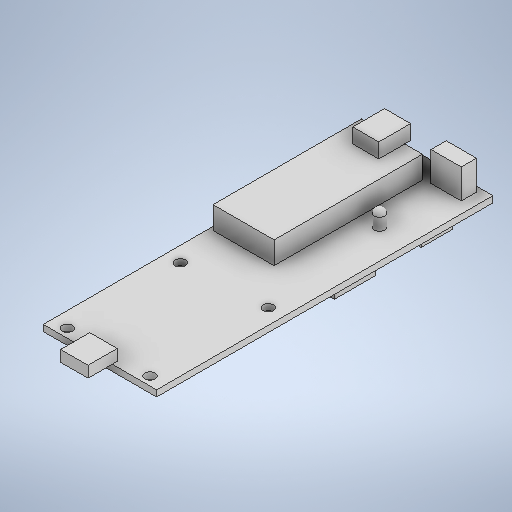
# Autodesk Inventor part: PCB Board
Saved by Autodesk Inventor 2025 (Build 290162000, 162)
## iProperties
Created: 2024-07-09
Part Number: PCB Board
Material: Generic
Document SubType Name: Modeling
Designer: track
Density: 1 g/cm^3
Appearance: Default
Author: track
Autodesk Inventor part; units mm, degrees
ref_plane "YZ Plane" through (0, 0, 0) normal (1, 0, 0) x (0, 1, 0)
ref_plane "XZ Plane" through (0, 0, 0) normal (0, 1, 0) x (-1, 0, 0)
ref_plane "XY Plane" through (0, 0, 0) normal (0, 0, 1) x (1, 0, 0)
sketch "Sketch1" plane through (0, 0, 0) normal (0, 1, 0) x (-1, 0, 0)
  line L0 (16.375, 48.6) -> (-16.375, 48.6)
  line L1 (-16.375, 48.6) -> (-16.375, -48.6)
  line L2 (-16.375, -48.6) -> (16.375, -48.6)
  line L3 (16.375, -48.6) -> (16.375, 48.6)
  line L4 (16.375, 48.6) -> (-16.375, -48.6) construction
  line L5 (-16.375, 48.6) -> (16.375, -48.6) construction
  point P0 (0, 0)
  dimension "d0" = 32.75
  dimension "d1" = 97.2
  constraints: 12 end point, 2 midpoint, 2 parallel, 1 horizontal, 1 perpendicular
  measures "d0" distance of L0.start L0.end
  measures "d1" distance of L0.end L1.end
extrude "Extrusion1" add sketch "Sketch1" along normal blind 1.8
sketch "Sketch4" plane through (0, 0, 0) normal (0, -1, 0) x (1, 0, 0)
  line L0 (8.375, 33.45) -> (-9.375, 33.45)
  line L1 (-9.375, 33.45) -> (-9.375, 15.45)
  line L2 (-9.375, 15.45) -> (8.375, 15.45)
  line L3 (8.375, 15.45) -> (8.375, 33.45)
  line L4 (16.375, 48.6) -> (16.375, -48.6) projected
  line L5 (-16.375, 48.6) -> (16.375, 48.6) projected
  point P0 (0, 0)
  dimension "d12" = 18
  dimension "d13" = 17.75
  dimension "d14" = 8
  dimension "d15" = 15.15
  constraints: 8 end point, 2 parallel, 1 horizontal, 1 perpendicular
  measures "d12" distance of L2.end L0.start
  measures "d13" distance of L1.end L2.end
  measures "d14" distance between parallel lines of L4 L3
  measures "d15" distance between parallel lines of L5 L0
extrude "Extrusion4" add sketch "Sketch4" along normal blind 3.43 from surface at -1.8
sketch "Sketch5" plane through (-9.375, -1.63, 33.45) normal (0, -1, 0) x (1, 0, 0)
  line L0 (2, -9) -> (15.8, -9)
  line L1 (15.8, -9) -> (15.8, 9.6)
  line L2 (15.8, 9.6) -> (2, 9.6)
  line L3 (2, 9.6) -> (2, -9)
  line L4 (0, 0) -> (0, -18) projected
  line L5 (0, -18) -> (17.75, -18) projected
  point P0 (9.375, -33.45)
  dimension "d18" = 18.6
  dimension "d19" = 13.8
  dimension "d20" = 2
  dimension "d21" = 9
  constraints: 8 end point, 2 parallel, 1 horizontal, 1 perpendicular
  measures "d18" distance of L0.end L1.end
  measures "d19" distance of L1.end L2.end
  measures "d20" distance between parallel lines of L4 L3
  measures "d21" distance between parallel lines of L5 L0
extrude "Extrusion5" add sketch "Sketch5" along normal blind 1.75 from surface at 0
sketch "Sketch6" plane through (0, 0, 0) normal (0, -1, 0) x (1, 0, 0)
  line L0 (14.375, -4.75) -> (3.525, -4.75)
  line L1 (3.525, -4.75) -> (3.525, -16.6)
  line L2 (3.525, -16.6) -> (14.375, -16.6)
  line L3 (14.375, -16.6) -> (14.375, -4.75)
  line L4 (16.375, 48.6) -> (16.375, -48.6) projected
  line L5 (16.375, -48.6) -> (-16.375, -48.6) projected
  point P0 (0, 0)
  dimension "d24" = 11.85
  dimension "d25" = 10.85
  dimension "d26" = 2
  dimension "d27" = 32
  constraints: 8 end point, 2 parallel, 1 horizontal, 1 perpendicular
  measures "d24" distance of L2.end L0.start
  measures "d25" distance of L1.end L2.end
  measures "d26" distance between parallel lines of L4 L3
  measures "d27" distance between parallel lines of L5 L2
extrude "Extrusion6" add sketch "Sketch6" along normal blind 5.04 from surface at -1.8
sketch "Sketch7" plane through (0, 0, 0) normal (0, -1, 0) x (1, 0, 0)
  line L0 (14.775, -29.45) -> (4.445, -29.45)
  line L1 (4.445, -29.45) -> (4.445, -38.6)
  line L2 (4.445, -38.6) -> (14.775, -38.6)
  line L3 (14.775, -38.6) -> (14.775, -29.45)
  line L4 (16.375, 48.6) -> (16.375, -48.6) projected
  line L5 (16.375, -48.6) -> (-16.375, -48.6) projected
  point P0 (0, 0)
  dimension "d30" = 9.15
  dimension "d31" = 10.33
  dimension "d32" = 1.6
  dimension "d33" = 10
  constraints: 8 end point, 2 parallel, 1 horizontal, 1 perpendicular
  measures "d30" distance of L2.end L0.start
  measures "d31" distance of L1.end L2.end
  measures "d32" distance between parallel lines of L4 L3
  measures "d33" distance between parallel lines of L5 L2
extrude "Extrusion7" add sketch "Sketch7" along normal blind 4.18 from surface at -1.8
sketch "Sketch8" plane through (0, 1.8, 0) normal (0, 1, 0) x (1, 0, 0)
  line L0 (-4.375, -47.18) -> (3.555, -47.18)
  line L1 (3.555, -47.18) -> (3.555, -55.6)
  line L2 (3.555, -55.6) -> (-4.375, -55.6)
  line L3 (-4.375, -55.6) -> (-4.375, -47.18)
  line L4 (-16.375, 48.6) -> (-16.375, -48.6) projected
  line L5 (-16.375, -48.6) -> (16.375, -48.6) projected
  point P0 (0, 0)
  dimension "d36" = 8.42
  dimension "d37" = 7.93
  dimension "d38" = 12
  dimension "d39" = 7
  constraints: 8 end point, 2 parallel, 1 horizontal, 1 perpendicular
  measures "d36" distance of L2.end L0.start
  measures "d37" distance of L1.end L2.end
  measures "d38" distance between parallel lines of L4 L3
  measures "d39" distance between parallel lines of L5 L2
extrude "Extrusion8" add sketch "Sketch8" along normal blind 3.23
sketch "Sketch9" plane through (0, 1.8, 0) normal (0, 1, 0) x (1, 0, 0)
  circle A0 centre (-11.975, -46.1) radius 1.5
  circle A1 centre (11.975, -46.1) radius 1.5
  circle A2 centre (11.975, -11.9) radius 1.5
  circle A3 centre (-11.975, -13.4) radius 1.5
  line L0 (-13.475, -13.4) -> (-16.375, -13.4)
  line L1 (-16.375, 48.6) -> (-16.375, -48.6) projected
  line L2 (-13.475, -13.4) -> (-11.975, -13.4) construction
  line L3 (-11.975, -46.1) -> (-13.475, -46.1) construction
  line L4 (-13.475, -46.1) -> (-16.375, -46.1)
  line L5 (-11.975, -46.1) -> (-11.975, -47.6) construction
  line L6 (-16.375, -48.6) -> (16.375, -48.6) projected
  line L7 (-11.975, -47.6) -> (-11.975, -48.6)
  line L8 (11.975, -46.1) -> (13.475, -46.1) construction
  line L9 (13.475, -46.1) -> (16.375, -46.1)
  line L10 (11.975, -46.1) -> (11.975, -47.6) construction
  line L11 (11.975, -47.6) -> (11.975, -48.6)
  line L12 (16.375, -48.6) -> (16.375, 48.6) projected
  line L13 (11.975, -46.1) -> (11.975, -44.6) construction
  line L14 (11.975, -44.6) -> (11.975, -13.4)
  line L15 (11.975, -13.4) -> (11.975, -11.9) construction
  line L16 (-11.975, -46.1) -> (-11.975, -14.9)
  line L17 (-11.975, -13.4) -> (-11.975, -14.9) construction
  point P0 (0, 0)
  dimension "d42" = 3
  dimension "d43" = 2.9
  dimension "d44" = 2.9
  dimension "d45" = 1
  dimension "d46" = 1
  dimension "d47" = 2.9
  dimension "d48" = 31.2
  dimension "d49" = 31.2
  constraints: 30 end point, 9 point on line, 7 point on circle, 4 horizontal, 4 vertical, 3 centre point, 2 equal radius, 2 perpendicular, 1 vertical alignment, 3 other
  measures "d42" diameter of A0
  measures "d43" distance of L0.start L0.end
  measures "d44" distance of L3.end L4.end
  measures "d45" distance of L5.end L7.end
  measures "d46" distance of L10.end L11.end
  measures "d47" distance of L8.end L9.end
  measures "d48" distance of L13.end L14.end
  measures "d49" distance of L3.start L16.end
extrude "Extrusion9" cut sketch "Sketch9" against normal through all contours A0 | A2 | A3 | A1
sketch "Sketch10" plane through (0, 1.8, 0) normal (0, 1, 0) x (1, 0, 0)
  line L0 (2.275, -0.55) -> (-15.375, -0.55)
  line L1 (-15.375, -0.55) -> (-15.375, 42.35)
  line L2 (-15.375, 42.35) -> (2.275, 42.35)
  line L3 (2.275, 42.35) -> (2.275, -0.55)
  line L4 (-16.375, 48.6) -> (-16.375, -48.6) projected
  line L5 (16.375, 48.6) -> (-16.375, 48.6) projected
  point P0 (0, 0)
  dimension "d52" = 42.9
  dimension "d53" = 17.65
  dimension "d54" = 1
  dimension "d55" = 6.25
  constraints: 8 end point, 2 parallel, 1 horizontal, 1 perpendicular
  measures "d52" distance of L0.end L1.end
  measures "d53" distance of L0.start L0.end
  measures "d54" distance between parallel lines of L4 L1
  measures "d55" distance between parallel lines of L5 L2
extrude "Extrusion10" add sketch "Sketch10" along normal blind 6.45
sketch "Sketch11" plane through (0, 8.25, 0) normal (0, 1, 0) x (1, 0, 0)
  line L0 (-10.375, 34.85) -> (-2.855, 34.85)
  line L1 (-2.855, 34.85) -> (-2.855, 44.05)
  line L2 (-2.855, 44.05) -> (-10.375, 44.05)
  line L3 (-10.375, 44.05) -> (-10.375, 34.85)
  line L4 (2.275, 42.35) -> (-15.375, 42.35) projected
  line L5 (-15.375, 42.35) -> (-15.375, -0.55) projected
  point P0 (0, 0)
  dimension "d58" = 9.2
  dimension "d59" = 7.52
  dimension "d60" = 7.5
  dimension "d61" = 5
  constraints: 8 end point, 2 parallel, 1 horizontal, 1 perpendicular
  measures "d58" distance of L2.end L0.start
  measures "d59" distance of L1.end L2.end
  measures "d60" distance between parallel lines of L4 L0
  measures "d61" distance between parallel lines of L5 L3
extrude "Extrusion11" add sketch "Sketch11" along normal blind 4.25
sketch "Sketch12" plane through (0, 1.8, 0) normal (0, 1, 0) x (1, 0, 0)
  circle A0 centre (7.875, 24.35) radius 1.5
  line L0 (7.875, 24.35) -> (9.375, 24.35) construction
  line L1 (9.375, 24.35) -> (16.375, 24.35)
  line L2 (16.375, -48.6) -> (16.375, 48.6) projected
  line L3 (7.875, 24.35) -> (7.875, 25.85) construction
  line L4 (7.875, 25.85) -> (7.875, 48.6)
  line L5 (16.375, 48.6) -> (-16.375, 48.6) projected
  point P0 (0, 0)
  dimension "d64" = 3
  dimension "d65" = 7
  dimension "d66" = 22.75
  constraints: 8 end point, 4 point on line, 2 point on circle, 1 centre point, 1 horizontal, 1 vertical
  measures "d64" diameter of A0
  measures "d65" distance of L0.end L1.end
  measures "d66" distance of L3.end L4.end
extrude "Extrusion12" add sketch "Sketch12" along normal blind 5 contours A0
fillet "Fillet1" radius 1.5 1 edges at (6.375, 6.8, -24.35)
sketch "Sketch13" plane through (0, 1.8, 0) normal (0, 1, 0) x (1, 0, 0)
  line L0 (13.125, 47.1) -> (4.375, 47.1)
  line L1 (4.375, 47.1) -> (4.375, 42.7)
  line L2 (4.375, 42.7) -> (13.125, 42.7)
  line L3 (13.125, 42.7) -> (13.125, 47.1)
  line L4 (16.375, 48.6) -> (-16.375, 48.6) projected
  line L5 (16.375, -48.6) -> (16.375, 48.6) projected
  point P0 (0, 0)
  dimension "d70" = 8.75
  dimension "d71" = 4.4
  dimension "d72" = 1.5
  dimension "d73" = 3.25
  constraints: 8 end point, 2 parallel, 1 horizontal, 1 perpendicular
  measures "d70" distance of L0.start L0.end
  measures "d71" distance of L0.end L1.end
  measures "d72" distance between parallel lines of L4 L0
  measures "d73" distance between parallel lines of L5 L3
extrude "Extrusion13" add sketch "Sketch13" along normal blind 10.3 from surface at -1.8
body "Solid1"
